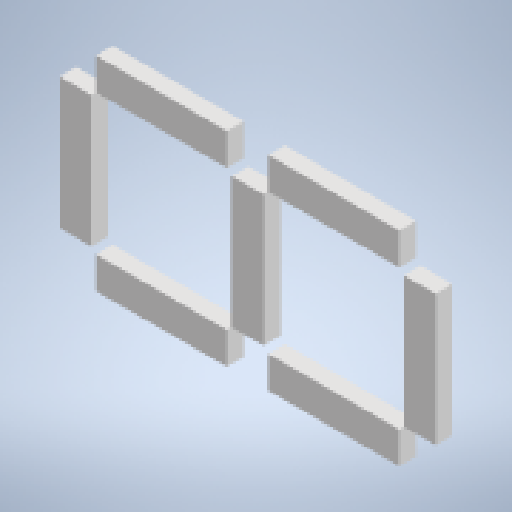
# Autodesk Inventor part: Digit
Saved by Autodesk Inventor 2024.2 (Build 282272000, 272)
## iProperties
Created: 2024-01-22
Part Number: Digit
Material: Generic
Document SubType Name: Modeling
Designer: Felix
Density: 1 g/cm^3
Appearance: Default
Author: Felix
Autodesk Inventor part; units mm, degrees
ref_plane "YZ Plane" through (0, 0, 0) normal (1, 0, 0) x (0, 1, 0)
ref_plane "XZ Plane" through (0, 0, 0) normal (0, 1, 0) x (-1, 0, 0)
ref_plane "XY Plane" through (0, 0, 0) normal (0, 0, 1) x (1, 0, 0)
sketch "Sketch1" plane through (0, 0, 0) normal (0, 1, 0) x (-1, 0, 0)
  line L0 (92, 46) -> (0, 46) construction
  line L1 (0, 46) -> (0, -46) construction
  line L2 (0, -46) -> (92, -46) construction
  line L3 (92, -46) -> (92, 46) construction
  line L4 (0, 46) -> (-92, 46) construction
  line L5 (-92, 46) -> (-92, -46) construction
  line L6 (-92, -46) -> (0, -46) construction
  line L7 (0, -46) -> (0, 46) construction
  line L8 (81, 54.5) -> (11, 54.5)
  line L9 (11, 54.5) -> (11, 37.5)
  line L10 (11, 37.5) -> (81, 37.5)
  line L11 (81, 37.5) -> (81, 54.5)
  line L12 (8.5, 35) -> (-8.5, 35)
  line L13 (-8.5, 35) -> (-8.5, -35)
  line L14 (-8.5, -35) -> (8.5, -35)
  line L15 (8.5, -35) -> (8.5, 35)
  line L16 (92, 0) -> (-92, 0) construction
  line L17 (46, 46) -> (46, -46) construction
  line L18 (83.5, 35) -> (100.5, 35)
  line L19 (100.5, 35) -> (100.5, -35)
  line L20 (100.5, -35) -> (83.5, -35)
  line L21 (83.5, -35) -> (83.5, 35)
  line L22 (-46, 46) -> (-46, -46) construction
  line L23 (-100.5, 35) -> (-83.5, 35)
  line L24 (-83.5, 35) -> (-83.5, -35)
  line L25 (-83.5, -35) -> (-100.5, -35)
  line L26 (-100.5, -35) -> (-100.5, 35)
  line L27 (-81, 54.5) -> (-11, 54.5)
  line L28 (-11, 54.5) -> (-11, 37.5)
  line L29 (-11, 37.5) -> (-81, 37.5)
  line L30 (-81, 37.5) -> (-81, 54.5)
  line L31 (81, -54.5) -> (11, -54.5)
  line L32 (11, -54.5) -> (11, -37.5)
  line L33 (11, -37.5) -> (81, -37.5)
  line L34 (81, -37.5) -> (81, -54.5)
  line L35 (-11, -54.5) -> (-11, -37.5)
  line L36 (-11, -37.5) -> (-81, -37.5)
  line L37 (-81, -54.5) -> (-11, -54.5)
  line L38 (-81, -37.5) -> (-81, -54.5)
  point P0 (0, 0)
  point P1 (0, 0)
  point P2 (81, 46)
  point P3 (0, 35)
  point P4 (92, 35)
  point P5 (-92, 0)
  point P6 (-92, 35)
  point P7 (-81, 46)
  point P8 (81, -46)
  point P9 (-81, -46)
  dimension "d2" = 92
  dimension "d3" = 92
  dimension "d4" = 17
  dimension "d5" = 17
  dimension "d6" = 70
  dimension "d7" = 70
  dimension "d8" = 92
  constraints: 78 end point, 27 symmetric about line, 9 midpoint, 8 parallel, 4 horizontal, 4 perpendicular, 3 coincident, 3 point on line, 2 other
  measures "d2" distance of L2.end L0.start
  measures "d3" distance of L0.end L4.end
  measures "d4" distance of L10.end L8.start
  measures "d5" distance of L12.start L12.end
  measures "d6" distance of L8.start L8.end
  measures "d7" distance of L14.end L12.start
  measures "d8" distance of L0.start L0.end
extrude "Extrusion1" add sketch "Sketch1" along normal blind 9
equation "\"d2\" = d8"
equation "\"d3\" = d8"
equation "\"d5\" = d4"
equation "\"d7\" = d6"
body "Solid1"
